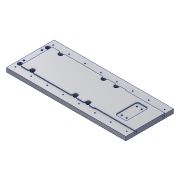
# Autodesk Inventor part: Grundplatte
Saved by Autodesk Inventor 2016 (Build 200138000, 138)
## iProperties
Created: 2015-07-27
Part Number: Grundplatte
Material: Aluminum 6061
Document SubType Name: Modeling
Density: 2.7 g/cm^3
Appearance: Aluminum - Flat
Autodesk Inventor part; units mm, degrees
ref_plane "YZ Plane" through (0, 0, 0) normal (1, 0, 0) x (0, 1, 0)
ref_plane "XZ Plane" through (0, 0, 0) normal (0, 1, 0) x (-1, 0, 0)
ref_plane "XY Plane" through (0, 0, 0) normal (0, 0, 1) x (1, 0, 0)
sketch "Sketch1" plane through (0, 0, 0) normal (0, 0, 1) x (1, 0, 0)
  line L0 (-150, -60) -> (150, -60)
  line L1 (150, -60) -> (150, 60)
  line L2 (150, 60) -> (-150, 60)
  line L3 (-150, 60) -> (-150, -60)
  line L4 (-150, -60) -> (150, 60) construction
  line L5 (150, -60) -> (-150, 60) construction
  point P0 (0, 0)
  dimension "d0" = 300
  dimension "d1" = 120
  constraints: 12 end point, 2 midpoint, 2 parallel, 1 horizontal, 1 perpendicular
  measures "d0" distance of L2.end L1.end
  measures "d1" distance of L1.end L0.end
extrude "Extrusion1" add sketch "Sketch1" along normal blind 12
sketch "Sketch2" plane through (0, 0, 12) normal (0, 0, 1) x (1, 0, 0)
  line L0 (150, -60) -> (-150, -60)
  line L1 (-150, -60) -> (-150, -40)
  line L2 (-150, -40) -> (150, -40)
  line L3 (150, -40) -> (150, -60)
  line L4 (150, 60) -> (-150, 60)
  line L5 (-150, 60) -> (-150, 40)
  line L6 (-150, 40) -> (150, 40)
  line L7 (150, 40) -> (150, 60)
  line L8 (-135, 40) -> (-150, 40)
  line L9 (-150, 40) -> (-150, -40)
  line L10 (-150, -40) -> (-135, -40)
  line L11 (-135, -40) -> (-135, 40)
  line L12 (150, -60) -> (150, 60) projected
  line L13 (-150, -60) -> (150, -60) projected
  line L14 (-150, 60) -> (-150, -60) projected
  line L15 (150, 60) -> (-150, 60) projected
  line L16 (119, 28) -> (91, 28)
  line L17 (91, 28) -> (91, -28)
  line L18 (91, -28) -> (119, -28)
  line L19 (119, -28) -> (119, 28)
  line L20 (150, -40) -> (50, -40)
  line L21 (50, -40) -> (50, -38)
  line L22 (50, -38) -> (150, -38)
  line L23 (150, -38) -> (150, -40)
  line L24 (150, 40) -> (50, 40)
  line L25 (50, 40) -> (50, 38)
  line L26 (50, 38) -> (150, 38)
  line L27 (150, 38) -> (150, 40)
  point P0 (0, 0)
  point P1 (91, 0)
  dimension "d4" = 80
  dimension "d5" = 15
  dimension "d6" = 269
  dimension "d7" = 28
  dimension "d8" = 56
  dimension "d25" = 100
  dimension "d26" = 2
  constraints: 48 end point, 12 parallel, 9 collinear, 6 horizontal, 6 perpendicular, 1 horizontal alignment, 1 midpoint, 1 point on line
  measures "d4" distance between parallel lines of L6 L2
  measures "d5" distance between parallel lines of L9 L11
  measures "d6" distance between parallel lines of L14 L19
  measures "d7" distance of L17.end L18.end
  measures "d8" distance of L18.end L16.start
  measures "d25" distance of L21.end L22.end
  measures "d26" distance of L20.end L21.end
extrude "Extrusion2" cut sketch "Sketch2" against normal blind 2 contours L0 L1 L2 L3 | L2 L21 L22 L12 | L9 L6 L11 L2 | L5 L4 L7 L6 | L26 L25 L6 L12 | L19 L18 L17 L16
fillet "Fillet1" radius 5 4 edges at (119, 28, 11) (91, 28, 11) (91, -28, 11) (119, -28, 11)
sketch "Sketch3" plane through (0, 0, 12) normal (0, 0, 1) x (1, 0, 0)
  line L0 (-150, -60) -> (-150, 60) projected
  point P0 (0, 0)
  point P1 (-141, -35)
  point P2 (-109, -35)
  point P3 (-109, 35)
  point P4 (-141, 35)
  point P5 (-1, -35)
  point P6 (31, -35)
  point P7 (31, 35)
  point P8 (-1, 35)
  dimension "d12" = 32
  dimension "d13" = 32
  dimension "d14" = 172
  dimension "d15" = 70
  dimension "d16" = 9
  dimension "d17" = 35
  constraints: 6 horizontal alignment, 4 vertical alignment
  measures "d12" distance of point (-109, -35) point (-141, -35)
  measures "d13" distance of point (31, -35) point (-1, -35)
  measures "d14" distance of point (-141, -35) point (31, -35)
  measures "d15" distance of point (-141, 35) point (-141, -35)
  measures "d16" distance from line of L0 point (-141, -35)
  measures "d17" vertical distance of point (0, 0) point (-141, -35)
hole "Hole1" at (-141, -35, 12) at (-109, -35, 12) at (-109, 35, 12) at (-141, 35, 12) at (-1, -35, 12) at (31, -35, 12) at (31, 35, 12) at (-1, 35, 12) direction (0, 0, -1) diameter 5.5 end through all counterbore diameter 10 counterbore depth 7.7 clearance for "Socket Head Cap Screw ISO 4762" size "M5" standard "ISO"
fillet "Fillet2" radius 3 2 edges at (50, 38, 11) (50, -38, 11)
sketch "Sketch4" plane through (0, 0, 12) normal (0, 0, 1) x (1, 0, 0)
  circle A0 centre (-109, -35) radius 5 projected
  line L0 (-104, -35) -> (-104, -40)
  line L1 (-104, -40) -> (-114, -40)
  line L2 (-114, -40) -> (-114, -35)
  line L3 (-135, -40) -> (-109, -40) projected
  circle A1 centre (-1, -35) radius 5 projected
  circle A2 centre (31, -35) radius 5 projected
  line L4 (36, -35) -> (36, -40)
  line L5 (36, -40) -> (26, -40)
  line L6 (26, -40) -> (26, -35)
  line L7 (4, -35) -> (4, -40)
  line L8 (4, -40) -> (-6, -40)
  line L9 (-6, -40) -> (-6, -35)
  line L10 (-1, -40) -> (31, -40) projected
  point P0 (0, 0)
  constraints: 18 end point, 6 point on circle, 6 tangent, 5 vertical, 2 collinear, 2 perpendicular, 2 point on line, 1 parallel
extrude "Extrusion3" cut sketch "Sketch4" against normal up to surface (2 mm away) contours L0 L1 A0 | A0 L1 L2 | L7 L8 A1 | A1 L8 L9 | L4 L5 A2 | A2 L5 L6
mirror "Mirror1" about plane through (0, 0, 0) normal (0, 1, 0) of "Extrusion3"
fillet "Fillet3" radius 3 14 edges at (-135, 40, 11) (-135, -40, 11) (36, 40, 11) (26, 40, 11) (4, 40, 11) (-6, 40, 11) (-104, 40, 11) (-114, 40, 11) (-114, -40, 11) (-104, -40, 11) (-6, -40, 11) (4, -40, 11) (26, -40, 11) (36, -40, 11)
sketch "Sketch5" plane through (0, 0, 10) normal (0, 0, 1) x (1, 0, 0)
  line L0 (-150, -60) -> (-150, 60) projected
  line L1 (-117, 40) -> (-132, 40) projected
  point P0 (0, 0)
  point P1 (-140, 47.5)
  dimension "d31" = 10
  dimension "d32" = 7.5
  measures "d31" distance from line of L0 point (-140, 47.5)
  measures "d32" distance from line of point (-140, 47.5) L1
hole "Hole2" at (-140, 47.5, 10) direction (0, 0, -1) diameter 2.459 end through all thread size "M3x0.5" designation "M3" class "6H" standard "ISO Metric profile"
pattern_linear "Rectangular Pattern1" count 8 spacing 40 along (1, 0, 0) of "Hole2"
mirror "Mirror2" about plane through (0, 0, 0) normal (0, 1, 0) of "Hole2", "Rectangular Pattern1"
sketch "Sketch6" plane through (150, -60, 0) normal (1, 0, 0) x (0, 0, -1)
  line L0 (0, 0) -> (0, 120) projected
  point P0 (0, 60)
  point P1 (-6, 25)
  point P2 (-6, 95)
  dimension "d43" = 70
  dimension "d44" = 35
  dimension "d45" = 6
  constraints: 1 vertical alignment
  measures "d43" distance of point (-6, 95) point (-6, 25)
  measures "d44" vertical distance of point (0, 60) point (-6, 25)
  measures "d45" distance from line of L0 point (-6, 25)
hole "Hole3" at (150, -35, 6) at (150, 35, 6) direction (-1, 0, 0) diameter 4.917 depth 20 tip angle 118 thread size "M6x1" designation "M6" class "6H" standard "ISO Metric profile"
sketch "Sketch7" plane through (0, 0, 10) normal (0, 0, 1) x (1, 0, 0)
  line L0 (-150, -60) -> (-150, 60) projected
  line L1 (-117, 40) -> (-132, 40) projected
  line L2 (-132, -40) -> (-117, -40) projected
  point P0 (0, 0)
  point P1 (-143, 22.5)
  point P2 (-143, -23)
  dimension "d53" = 45.5
  dimension "d54" = 7
  dimension "d55" = 17.5
  dimension "d56" = 17
  constraints: 1 vertical alignment
  measures "d53" distance of point (-143, -23) point (-143, 22.5)
  measures "d54" distance from line of point (-143, 22.5) L0
  measures "d55" distance from line of L1 point (-143, 22.5)
  measures "d56" distance from line of L2 point (-143, -23)
hole "Hole4" at (-143, 22.5, 10) at (-143, -23, 10) direction (0, 0, -1) diameter 4.134 end through all thread size "M5x0.8" designation "M5" class "6H" standard "ISO Metric profile"
sketch "Sketch8" plane through (0, 0, 10) normal (0, 0, 1) x (1, 0, 0)
  line L0 (99, 19) -> (111, 19)
  line L1 (111, 19) -> (111, -19)
  line L2 (111, -19) -> (99, -19)
  line L3 (99, -19) -> (99, 19)
  line L4 (99, 19) -> (111, -19) construction
  line L5 (111, 19) -> (99, -19) construction
  line L6 (91, -23) -> (91, 23) projected
  point P0 (0, 0)
  point P1 (105, 0)
  point P2 (105, 0)
  dimension "d64" = 38
  dimension "d65" = 12
  dimension "d66" = 8
  constraints: 12 end point, 3 midpoint, 2 parallel, 1 horizontal, 1 horizontal alignment, 1 perpendicular
  measures "d64" distance of L2.end L0.start
  measures "d65" distance of L0.start L0.end
  measures "d66" distance between parallel lines of L6 L3
hole "Hole5" at (111, 19, 10) at (99, 19, 10) at (99, -19, 10) at (111, -19, 10) direction (0, 0, -1) diameter 3.242 end through all thread size "M4x0.7" designation "M4" class "6H" standard "ISO Metric profile"
equation "\"d17\" = 0.5 * d15"
equation "\"d44\" = 0.5 * d43"
body "Solid1"
